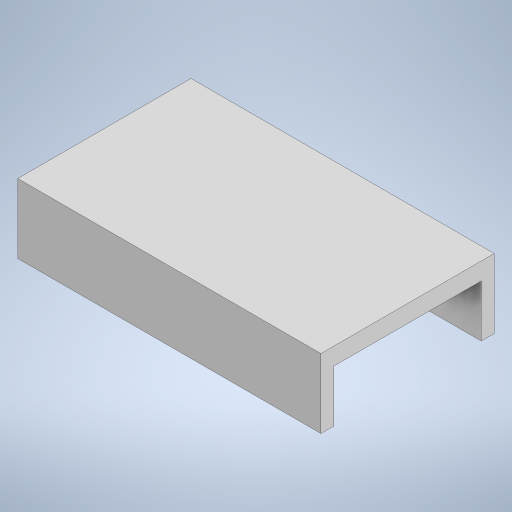
# Autodesk Inventor part: Battery box under the board
Saved by Autodesk Inventor 2023 (Build 270158000, 158)
## iProperties
Created: 2023-05-22
Part Number: Battery box under the board
Material: Типовые
Document SubType Name: Modeling
Designer: ivanc
Density: 1 g/cm^3
Appearance: По умолчанию
Author: ivanc
Autodesk Inventor part; units mm, degrees
ref_plane "YZ Plane" through (0, 0, 0) normal (1, 0, 0) x (0, 1, 0)
ref_plane "XZ Plane" through (0, 0, 0) normal (0, 1, 0) x (-1, 0, 0)
ref_plane "XY Plane" through (0, 0, 0) normal (0, 0, 1) x (1, 0, 0)
sketch "Эскиз1" plane through (0, 0, 0) normal (0, 1, 0) x (-1, 0, 0)
  line L0 (-35, 20) -> (35, 20)
  line L1 (35, 20) -> (35, -20)
  line L2 (35, -20) -> (-35, -20)
  line L3 (-35, -20) -> (-35, 20)
  line L4 (-35, 20) -> (35, -20) construction
  line L5 (35, 20) -> (-35, -20) construction
  point P0 (0, 0)
  dimension "d0" = 40
  dimension "d1" = 70
  constraints: 12 end point, 2 midpoint, 2 parallel, 1 horizontal, 1 perpendicular
  measures "d0" distance of L0.end L1.end
  measures "d1" distance of L1.end L2.end
extrude "Выдавливание1" add sketch "Эскиз1" along normal blind 4
sketch "Эскиз2" plane through (0, 0, 0) normal (0, -1, 0) x (1, 0, 0)
  line L0 (-35, 20) -> (35, 20) projected
  line L1 (35, 20) -> (-35, 20)
  line L2 (-35, 20) -> (-35, 17)
  line L3 (-35, 17) -> (35, 17)
  line L4 (35, 17) -> (35, 20)
  line L5 (35, -20) -> (-35, -20) projected
  line L6 (35, -20) -> (-35, -20)
  line L7 (-35, -20) -> (-35, -17)
  line L8 (-35, -17) -> (35, -17)
  line L9 (35, -17) -> (35, -20)
  line L10 (-35, -20) -> (-35, 20) projected
  line L11 (-35, 17) -> (-32, 17)
  line L12 (-32, 17) -> (-32, -17)
  line L13 (-32, -17) -> (-35, -17)
  line L14 (-35, -17) -> (-35, 17)
  point P0 (0, 0)
  dimension "d4" = 3
  constraints: 24 end point, 6 parallel, 3 collinear, 3 horizontal, 3 perpendicular, 2 equal length
  measures "d4" distance of L3.end L0.end
extrude "Выдавливание2" add sketch "Эскиз2" along normal blind 12
